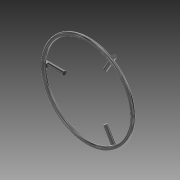
# Autodesk Inventor part: Kern
Saved by Autodesk Inventor 2014 (Build 180170000, 170)
## iProperties
Created: 2015-03-26
Part Number: Kern
Material: Silicon Nitride
Document SubType Name: Modeling
Designer: MSI
Density: 3.18 g/cm^3
Appearance: Chrome - Polished Black
Author: MSI
Autodesk Inventor part; units mm, degrees
ref_plane "XY Plane" through (0, 0, 0) normal (0, 0, 1) x (1, 0, 0)
sketch "Sketch1" plane through (0, 0, 0) normal (0, 0, 1) x (1, 0, 0)
  circle A0 centre (0, 0) radius 3
  line L0 (74, 5) -> (74, -5) construction
  point P0 (74, 0)
  dimension "d0" = 6
  dimension "d1" = 148
  dimension "d2" = 10
  constraints: 2 end point, 1 centre point, 1 coincident, 1 horizontal alignment, 1 midpoint, 1 vertical
  measures "d0" diameter of A0
  measures "d1" diameter of point (0, 0) L0
  measures "d2" distance of L0.start L0.end
revolve "Revolution1" add sketch "Sketch1" angle 360 about axis through (74, 5, 0) along (0, -1, 0)
ref_plane "Work Plane1" through (-3, 0, 0) normal (1, 0, 0) x (0, 1, 0)
sketch "Sketch2" plane through (-3, 0, 0) normal (1, 0, 0) x (0, 1, 0)
  circle A0 centre (6, 0) radius 3
  line L0 (6, 3) -> (0, 3)
  line L1 (0, 3) -> (0, -3)
  line L2 (0, -3) -> (6, -3)
  point P0 (0, 0)
  dimension "d5" = 6
  dimension "d6" = 6
  dimension "d7" = 6
  dimension "d8" = 6
  constraints: 6 end point, 2 point on circle, 2 tangent, 1 centre point, 1 horizontal, 1 horizontal alignment, 1 perpendicular
  measures "d5" diameter of A0
  measures "d6" distance of point (0, 0) A0.centre
  measures "d7" distance of L0.start L0.end
  measures "d8" distance of L0.end L1.end
extrude "Extrusion1" add sketch "Sketch2" along normal blind 6
sketch "Sketch3" plane through (3, 0, 0) normal (1, 0, 0) x (0, 0, -1)
  arc A0 (3, 6) -> (-3, 6) centre (0, 6) ccw projected
  circle A1 centre (0, 6) radius 3
  dimension "d11" = 6
  constraints: 1 centre point, 1 coincident
  measures "d11" diameter of A1
extrude "Extrusion2" add sketch "Sketch3" along normal blind 26
pattern_circular "Circular Pattern1" count 3 over 360 about axis through (74, 0, 0) along (0, 1, 0) of "Extrusion1", "Extrusion2"
ref_plane "Work Plane2" through (0, 9, 0) normal (0, 1, 0) x (-1, 0, 0)
sketch "Sketch4" plane through (0, 9, 0) normal (0, 1, 0) x (-1, 0, 0)
  circle A0 centre (-74, 0) radius 45.5
  point P0 (0, 0)
  dimension "d18" = 91
  dimension "d19" = 74
  constraints: 1 centre point, 1 horizontal alignment
  measures "d18" diameter of A0
  measures "d19" distance of point (0, 0) A0.centre
extrude "Extrusion3" cut sketch "Sketch4" against normal blind 26
body "Solid1"
